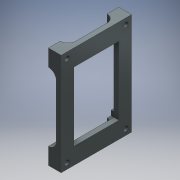
# Autodesk Inventor part: batteryholder
Saved by Autodesk Inventor 2016 (Build 200138000, 138)
## iProperties
Created: 2017-01-15
Part Number: batteryholder
Material: Generic
Document SubType Name: Modeling
Designer: hesaon
Density: 1 g/cm^3
Appearance: Default
Author: hesaon
Autodesk Inventor part; units mm, degrees
ref_plane "YZ Plane" through (0, 0, 0) normal (1, 0, 0) x (0, 1, 0)
ref_plane "XZ Plane" through (0, 0, 0) normal (0, 1, 0) x (-1, 0, 0)
ref_plane "XY Plane" through (0, 0, 0) normal (0, 0, 1) x (1, 0, 0)
sketch "Sketch1" plane through (0, 0, 0) normal (0, 1, 0) x (-1, 0, 0)
  line L0 (0, 0) -> (0, -104)
  line L1 (0, 0) -> (13, 0)
  line L2 (13, 0) -> (13, -12)
  line L3 (13, -12) -> (5, -12)
  line L4 (5, -12) -> (5, -92)
  line L5 (5, -92) -> (13, -92)
  line L6 (13, -92) -> (13, -104)
  line L7 (13, -104) -> (0, -104)
  dimension "d0" = 104
  dimension "d1" = 13
  dimension "d2" = 12
  dimension "d3" = 8
  dimension "d4" = 80
  dimension "d5" = 8
  constraints: 16 end point, 3 perpendicular, 2 point on line, 1 horizontal, 1 parallel, 1 vertical
  measures "d0" distance of L0.start L0.end
  measures "d1" distance of L0.start L1.end
  measures "d2" distance of L1.end L2.end
  measures "d3" distance of L2.end L3.end
  measures "d4" distance of L3.end L4.end
  measures "d5" distance of L4.end L5.end
extrude "Extrusion1" add sketch "Sketch1" along normal blind 72
sketch "Sketch3" plane through (-5, 0, -92) normal (-1, 0, 0) x (0, 0, 1)
  line L0 (0, 0) -> (80, 0) projected
  line L1 (0, 0) -> (80, 0) projected
  line L2 (80, 0) -> (80, 72) projected
  line L3 (0, 72) -> (80, 72) projected
  line L4 (0, 0) -> (0, 72) projected
  line L5 (0, 0) -> (0, 72) projected
  line L6 (80, 0) -> (0, 0)
  line L7 (0, 0) -> (0, 8)
  line L8 (0, 8) -> (80, 8)
  line L9 (80, 8) -> (80, 0)
  line L10 (80, 0) -> (80, 72) projected
  line L11 (80, 72) -> (0, 72)
  line L12 (0, 72) -> (0, 64)
  line L13 (0, 64) -> (80, 64)
  line L14 (80, 64) -> (80, 72)
  point P0 (92, 0)
  dimension "d14" = 8
  dimension "d15" = 8
  constraints: 16 end point, 4 parallel, 2 horizontal, 2 perpendicular, 2 point on line
  measures "d14" distance of L6.end L7.end
  measures "d15" distance of L12.end L11.end
extrude "Extrusion3" add sketch "Sketch3" along normal blind 8 contours L4 L8 L2 L0 | L4 L3 L2 L13
sketch "Sketch4" plane through (-13, 0, -104) normal (-1, 0, 0) x (0, 0, 1)
  circle A0 centre (98, 66) radius 2.5
  line L0 (0, 72) -> (104, 72) projected
  line L1 (0, 0) -> (0, 72) projected
  line L2 (0, 0) -> (104, 0) projected
  line L3 (104, 0) -> (104, 72) projected
  line L4 (12, 64) -> (92, 64) projected
  line L5 (92, 8) -> (92, 64) projected
  line L6 (92, 8) -> (12, 8) projected
  line L7 (12, 8) -> (12, 64) projected
  circle A1 centre (6, 6) radius 2.5
  circle A2 centre (98, 6) radius 2.5
  circle A3 centre (6, 66) radius 2.5
  line L8 (0, 0) -> (0, 72) projected
  line L9 (104, 0) -> (104, 72) projected
  dimension "d18" = 5
  dimension "d19" = 6
  dimension "d20" = 6
  dimension "d25" = 5
  dimension "d31" = 5
  dimension "d32" = 5
  dimension "d37" = 6
  dimension "d38" = 6
  dimension "d46" = 6
  dimension "d47" = 6
  constraints: 4 centre point, 2 vertical alignment
  measures "d18" diameter of A0
  measures "d19" distance from line of L0 A0.centre
  measures "d20" distance from line of L5 A0.centre
  measures "d25" diameter of A1
  measures "d31" diameter of A2
  measures "d32" diameter of A3
  measures "d37" distance from line of L1 A3.centre
  measures "d38" distance from line of L0 A3.centre
  measures "d46" distance from line of L2 A1.centre
  measures "d47" distance from line of L2 A2.centre
extrude "Extrusion5" cut sketch "Sketch4" against normal through all contours A0 | A1 | A2 | A3
sketch "Sketch5" plane through (-5, 8, -92) normal (-1, 0, 0) x (0, 0, 1)
  line L0 (80, 0) -> (0, 0) projected
  line L1 (5, 5) -> (75, 5)
  line L2 (75, 5) -> (75, 51)
  line L3 (75, 51) -> (5, 51)
  line L4 (5, 51) -> (5, 5)
  line L5 (0, 0) -> (0, 56) projected
  line L6 (80, 56) -> (0, 56) projected
  line L7 (0, 0) -> (0, 56) projected
  line L8 (0, 0) -> (80, 0) projected
  line L9 (80, 0) -> (80, 56) projected
  line L10 (0, 56) -> (80, 56) projected
  line L11 (80, 0) -> (80, 56) projected
  point P0 (92, -8)
  dimension "d50" = 5
  dimension "d51" = 5
  dimension "d52" = 5
  dimension "d53" = 5
  constraints: 8 end point, 2 parallel, 1 horizontal, 1 perpendicular
  measures "d50" distance between parallel lines of L5 L4
  measures "d51" distance between parallel lines of L6 L3
  measures "d52" distance between parallel lines of L9 L2
  measures "d53" distance between parallel lines of L0 L1
extrude "Extrusion6" cut sketch "Sketch5" against normal through all contours L4 L3 L2 L1
sketch "Sketch6" plane through (-13, 0, -104) normal (-1, 0, 0) x (0, 0, 1)
  line L0 (92, 8) -> (92, 64) projected
  line L1 (92, 12) -> (104, 12)
  line L2 (104, 0) -> (104, 72) projected
  line L3 (92, 60) -> (104, 60)
  line L4 (12, 8) -> (12, 64) projected
  line L5 (12, 12) -> (0, 12)
  line L6 (0, 0) -> (0, 72) projected
  line L7 (12, 60) -> (0, 60)
  line L8 (0, 72) -> (104, 72) projected
  line L9 (0, 0) -> (104, 0) projected
  line L10 (0, 12) -> (0, 60)
  line L11 (12, 12) -> (12, 60)
  line L12 (92, 12) -> (92, 60)
  line L13 (104, 12) -> (104, 60)
  dimension "d56" = 12
  dimension "d57" = 12
  constraints: 16 end point, 12 point on line, 2 parallel, 1 collinear, 1 horizontal, 1 perpendicular, 1 vertical
  measures "d56" distance between parallel lines of L8 L3
  measures "d57" distance between parallel lines of L9 L1
extrude "Extrusion7" cut sketch "Sketch6" against normal blind 8 contours L0 L3 L2 L1 | L6 L7 L4 L5
fillet "Fillet1" radius 8 1 edges at (-5, 12, -98)
fillet "Fillet2" radius 8 1 edges at (-5, 60, -98)
fillet "Fillet3" radius 8 2 edges at (-5, 12, -6) (-5, 60, -6)
sketch "Sketch7" plane through (-13, 72, -104) normal (-1, 0, 0) x (0, 0, 1)
  line L0 (104, 0) -> (0, 0) projected
  line L1 (17, -72) -> (87, -72)
  line L2 (87, -72) -> (87, 0)
  line L3 (87, 0) -> (17, 0)
  line L4 (17, 0) -> (17, -72)
  line L5 (0, -72) -> (0, -60) projected
  point P0 (104, -72)
  dimension "d63" = 17
  dimension "d64" = 17
  dimension "d65" = 72
  constraints: 8 end point, 2 parallel, 1 horizontal, 1 perpendicular, 1 point on line
  measures "d63" distance of point (104, -72) L1.end
  measures "d64" distance from line of L5 L1.start
  measures "d65" distance of L2.end L1.end
extrude "Extrusion8" cut sketch "Sketch7" against normal blind 8
fillet "Fillet4" radius 8 4 edges at (-5, 4, -87) (-5, 68, -87) (-5, 4, -17) (-5, 68, -17)
body "Solid1"
